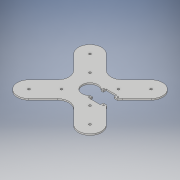
# Autodesk Inventor part: platform 1
Saved by Autodesk Inventor 2019 (Build 230136000, 136)
## iProperties
Created: 2019-02-09
Part Number: platform 1
Material: Generic
Document SubType Name: Modeling
Designer: mashi
Density: 1 g/cm^3
Appearance: Default
Author: mashi
Autodesk Inventor part; units mm, degrees
ref_plane "YZ Plane" through (0, 0, 0) normal (1, 0, 0) x (0, 1, 0)
ref_plane "XZ Plane" through (0, 0, 0) normal (0, 1, 0) x (-1, 0, 0)
ref_plane "XY Plane" through (0, 0, 0) normal (0, 0, 1) x (1, 0, 0)
sketch "Sketch1" plane through (0, 0, 0) normal (0, 1, 0) x (-1, 0, 0)
  circle A0 centre (0, 0) radius 120
  circle A1 centre (-9, 10) radius 1
  circle A2 centre (-9, -10) radius 1
  circle A3 centre (-29, -10) radius 1
  circle A4 centre (-29, 10) radius 1
  arc A5 (-8.0467, -7.5) -> (-8.0467, 7.5) centre (0, 0) ccw
  line L0 (-9, -7.5) -> (-8.0467, -7.5)
  line L1 (-9, -7.5) -> (-11, -7.5)
  line L2 (-11, -7.5) -> (-11, -11.5)
  line L3 (-29, -10) -> (-26, -10)
  line L4 (-11, -11.5) -> (-26, -11.5)
  line L5 (-26, -11.5) -> (-26, -7.5)
  line L6 (-26, -7.5) -> (-35, -7.5)
  line L7 (-35, -7.5) -> (-35, 0)
  line L8 (-9, 7.5) -> (-8.0467, 7.5)
  line L9 (-9, 7.5) -> (-11, 7.5)
  line L10 (-11, 7.5) -> (-11, 11.5)
  line L11 (-11, 11.5) -> (-26, 11.5)
  line L12 (-26, 11.5) -> (-26, 7.5)
  line L13 (-26, 7.5) -> (-35, 7.5)
  line L14 (-35, 7.5) -> (-35, 0)
  dimension "d0" = 240
  dimension "d5" = 2
  dimension "d6" = 2
  dimension "d7" = 2
  dimension "d8" = 2
  dimension "d9" = 22
  dimension "d12" = 2
  dimension "d13" = 3
  dimension "d14" = 4
  dimension "d15" = 9
  constraints: 30 end point, 6 centre point, 4 horizontal, 4 perpendicular, 2 coincident, 2 point on circle
  measures "d0" diameter of A0
  measures "d5" diameter of A1
  measures "d6" diameter of A2
  measures "d7" diameter of A3
  measures "d8" diameter of A4
  measures "d9" diameter of A5
  measures "d12" distance of L0.start L1.end
  measures "d13" distance of L3.start L3.end
  measures "d14" distance of L4.end L5.end
  measures "d15" distance of L5.end L6.end
extrude "Extrusion1" add sketch "Sketch1" along normal blind 2
sketch "Sketch4" plane through (0, 2, 0) normal (0, 1, 0) x (1, 0, 0)
  circle A0 centre (0, 0) radius 60
  circle A1 centre (0, 0) radius 120.1645
  dimension "d28" = 120
  dimension "d29" = 240.329
  constraints: 2 centre point, 2 coincident
  measures "d28" diameter of A0
  measures "d29" diameter of A1
extrude "Extrusion3" cut sketch "Sketch4" against normal blind 12
sketch "Sketch5" plane through (0, 2, 0) normal (0, 1, 0) x (1, 0, 0)
  circle A0 centre (0, 0) radius 28
  line L0 (0, 0) -> (19.799, 19.799)
  line L1 (0, 0) -> (28, 0) construction
  line L2 (19.799, 19.799) -> (-19.799, 19.799)
  line L3 (-19.799, 19.799) -> (-19.799, -19.799)
  line L4 (-19.799, -19.799) -> (19.799, -19.799)
  circle A1 centre (-19.799, -19.799) radius 3
  circle A2 centre (-19.799, 19.799) radius 3
  circle A3 centre (19.799, 19.799) radius 3
  circle A4 centre (19.799, -19.799) radius 3
  line L5 (19.799, 19.799) -> (42.4264, 42.4264)
  circle A5 centre (0, 0) radius 80
  circle A6 centre (0, 0) radius 60
  dimension "d56" = 56
  dimension "d57" = 45
  dimension "d58" = 6
  dimension "d59" = 6
  dimension "d60" = 6
  dimension "d62" = 6
  dimension "d63" = 32
  dimension "d64" = 160
  constraints: 12 end point, 7 centre point, 7 coincident, 4 point on circle, 2 horizontal, 2 point on line, 1 equal length, 1 perpendicular
  measures "d56" diameter of A0
  measures "d57" angle of L1 L0
  measures "d58" diameter of A1
  measures "d59" diameter of A2
  measures "d60" diameter of A3
  measures "d62" diameter of A4
  measures "d63" distance of L5.start L5.end
  measures "d64" diameter of A5
extrude "Extrusion4" add sketch "Sketch5" against normal blind 2 contours A5
sketch "Sketch8" plane through (0, 2, 0) normal (0, 1, 0) x (1, 0, 0)
  circle A0 centre (-42.4264, -42.4264) radius 3 projected
  arc A1 (-53.7401, -31.1127) -> (-31.1127, -53.7401) centre (-42.4264, -42.4264) ccw
  circle A2 centre (42.4264, -42.4264) radius 3 projected
  arc A3 (31.1127, -53.7401) -> (53.7401, -31.1127) centre (42.4264, -42.4264) ccw
  circle A4 centre (42.4264, 42.4264) radius 3 projected
  arc A5 (53.7401, 31.1127) -> (31.1127, 53.7401) centre (42.4264, 42.4264) ccw
  circle A6 centre (-42.4264, 42.4264) radius 3 projected
  arc A7 (-31.1127, 53.7401) -> (-53.7401, 31.1127) centre (-42.4264, 42.4264) ccw
  line L0 (-53.7401, 31.1127) -> (-33.9411, 11.3137)
  line L1 (11.3137, -33.9411) -> (31.1127, -53.7401)
  line L2 (-53.7401, -31.1127) -> (-33.9411, -11.3137)
  line L3 (11.3137, 33.9411) -> (31.1127, 53.7401)
  line L4 (-31.1127, 53.7401) -> (-11.3137, 33.9411)
  line L5 (33.9411, -11.3137) -> (53.7401, -31.1127)
  line L6 (-31.1127, -53.7401) -> (-11.3137, -33.9411)
  line L7 (33.9411, 11.3137) -> (53.7401, 31.1127)
  arc A8 (11.3137, -33.9411) -> (-11.3137, -33.9411) centre (0, -45.2548) ccw
  arc A9 (33.9411, 11.3137) -> (33.9411, -11.3137) centre (45.2548, 0) ccw
  arc A10 (-11.3137, 33.9411) -> (11.3137, 33.9411) centre (0, 45.2548) ccw
  arc A11 (-33.9411, -11.3137) -> (-33.9411, 11.3137) centre (-45.2548, 0) ccw
  circle A12 centre (0, 0) radius 80
  constraints: 16 end point, 16 point on circle, 14 tangent, 9 centre point, 5 coincident, 3 equal radius
extrude "Extrusion7" cut sketch "Sketch8" against normal blind 2 contours A12
sketch "Sketch10" plane through (0, 2, 0) normal (0, 1, 0) x (1, 0, 0)
  line L0 (0, 0) -> (60, 0) construction
  circle A0 centre (42.4264, -42.4264) radius 1.5
  circle A1 centre (19.799, -19.799) radius 1.5
  circle A2 centre (19.799, 19.799) radius 1.5
  circle A3 centre (42.4264, 42.4264) radius 1.5
  circle A4 centre (-19.799, 19.799) radius 1.5
  circle A5 centre (-42.4264, 42.4264) radius 1.5
  circle A6 centre (-19.799, -19.799) radius 1.5
  circle A7 centre (-42.4264, -42.4264) radius 1.5
  dimension "d128" = 3
  dimension "d129" = 3
  dimension "d132" = 360
  constraints: 8 centre point, 2 end point, 1 horizontal, 17 other
  measures "d128" diameter of A0
  measures "d129" diameter of A1
extrude "Extrusion9" cut sketch "Sketch10" against normal blind 10
body "Solid1"
